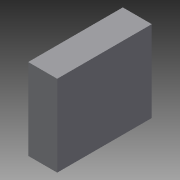
# Autodesk Inventor part: stig
Saved by Autodesk Inventor 2015 (Build 190159000, 159)
## iProperties
Created: 2015-10-09
Part Number: stig
Material: Generic
Description: insert part description/title
Document SubType Name: Modeling
Designer: c3132704
Density: 1 g/cm^3
Appearance: Default
Author: c3132704
Part Category: insert part category here and press enter to fill value
Autodesk Inventor part; units mm, degrees
ref_plane "YZ Plane" through (0, 0, 0) normal (1, 0, 0) x (0, 1, 0)
ref_plane "XZ Plane" through (0, 0, 0) normal (0, 1, 0) x (-1, 0, 0)
ref_plane "XY Plane" through (0, 0, 0) normal (0, 0, 1) x (1, 0, 0)
sketch "Sketch1" plane through (0, 0, 0) normal (1, 0, 0) x (0, 1, 0)
  line L0 (20.5035, 28.7943) -> (-60.9965, 28.7943)
  line L1 (-60.9965, 28.7943) -> (-60.9965, -41.2057)
  line L2 (-60.9965, -41.2057) -> (20.5035, -41.2057)
  line L3 (20.5035, -41.2057) -> (20.5035, 28.7943)
  point P0 (0, 0)
  dimension "d0" = 70
  dimension "d1" = 81.5
  constraints: 8 end point, 2 parallel, 1 horizontal, 1 perpendicular
  measures "d0" distance of L2.end L0.start
  measures "d1" distance of L1.end L2.end
extrude "Extrusion1" add sketch "Sketch1" along normal blind 25
body "Solid1"
